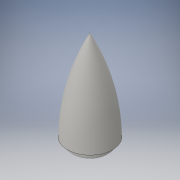
# Autodesk Inventor part: Rocket - Nose Cone
Saved by Autodesk Inventor 2016 (Build 200138000, 138)
## iProperties
Created: 2015-06-23
Part Number: Rocket - Nose Cone
Material: Generic
Document SubType Name: Modeling
Designer: The Shack
Density: 1 g/cm^3
Appearance: Default
Author: The Shack
Autodesk Inventor part; units mm, degrees
ref_plane "YZ Plane" through (0, 0, 0) normal (1, 0, 0) x (0, 1, 0)
ref_plane "XZ Plane" through (0, 0, 0) normal (0, 1, 0) x (-1, 0, 0)
ref_plane "XY Plane" through (0, 0, 0) normal (0, 0, 1) x (1, 0, 0)
sketch "Sketch1" plane through (0, 0, 0) normal (0, 0, 1) x (1, 0, 0)
  line L0 (0, 0) -> (-6.35, 0)
  line L1 (0, 0) -> (0, 25.4)
  spline S0 degree 2 poles (-6.35, 0) (-6.2585, 13.0686) (0, 25.4) knots 0 0 0 1 1 1
  point P0 (-4.7625, 12.7)
  dimension "d0" = 6.35
  dimension "d1" = 25.4
  constraints: 4 end point, 1 horizontal, 1 vertical, 3 other
  measures "d0" distance of L0.start L0.end
  measures "d1" distance of L0.start L1.end
revolve "Revolution1" add sketch "Sketch1" angle 360 about axis through (0, 0, 0) along (0, 1, 0)
sketch "Sketch2" plane through (0, 0, 0) normal (0, -1, 0) x (1, 0, 0)
  circle A0 centre (0, 0) radius 5.715
  dimension "d3" = 11.43
  constraints: 1 centre point, 1 coincident
  measures "d3" diameter of A0
extrude "Extrusion1" add sketch "Sketch2" along normal blind 2.54
fillet "Fillet1" radius 2.54 1 edges at (-5.715, -2.54, 0)
body "Solid1"
